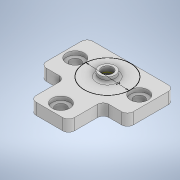
# Autodesk Inventor part: Pulley support
Saved by Autodesk Inventor 2022 (Build 260153000, 153)
## iProperties
Created: 2022-03-05
Part Number: Pulley support
Material: Genérico
Document SubType Name: Modeling
Designer: JK
Density: 1 g/cm^3
Appearance: Valor por defecto
Author: JK
Autodesk Inventor part; units mm, degrees
ref_plane "YZ Plane" through (0, 0, 0) normal (1, 0, 0) x (0, 1, 0)
ref_plane "XZ Plane" through (0, 0, 0) normal (0, 1, 0) x (-1, 0, 0)
ref_plane "XY Plane" through (0, 0, 0) normal (0, 0, 1) x (1, 0, 0)
sketch "Boceto1" plane through (0, 0, 0) normal (0, 1, 0) x (-1, 0, 0)
  circle A0 centre (0, 0) radius 12.15
  dimension "d0" = 24.3
  constraints: 1 centre point, 1 coincident
  measures "d0" diameter of A0
extrude "Extrusión1" add sketch "Boceto1" along normal blind 4
sketch "Boceto2" plane through (0, 0, 0) normal (0, -1, 0) x (1, 0, 0)
  line L0 (4.6765, 0) -> (2.3383, -4.05)
  line L1 (2.3383, -4.05) -> (-2.3383, -4.05)
  line L2 (-2.3383, -4.05) -> (-4.6765, 0)
  line L3 (-4.6765, 0) -> (-2.3383, 4.05)
  line L4 (-2.3383, 4.05) -> (2.3383, 4.05)
  line L5 (2.3383, 4.05) -> (4.6765, 0)
  circle A0 centre (0, 0) radius 4.05
  dimension "d3" = 8.1
  constraints: 12 end point, 2 coincident, 1 centre point, 1 tangent, 13 other
  measures "d3" diameter of A0
extrude "Extrusión2" cut sketch "Boceto2" against normal blind 4
sketch "Boceto3" plane through (0, 4, 0) normal (0, 1, 0) x (1, 0, 0)
  line L0 (2.3383, 4.05) -> (4.6765, 0) projected
  line L1 (4.6765, 0) -> (2.3383, -4.05) projected
  line L2 (2.3383, -4.05) -> (-2.3383, -4.05) projected
  line L3 (-2.3383, -4.05) -> (-4.6765, 0) projected
  line L4 (-4.6765, 0) -> (-2.3383, 4.05) projected
  line L5 (-2.3383, 4.05) -> (2.3383, 4.05) projected
  circle A0 centre (0, 0) radius 12.15 projected
  circle A1 centre (0, 0) radius 2.9
  dimension "d6" = 5.8
  constraints: 1 centre point, 1 coincident
  measures "d6" diameter of A1
extrude "Extrusión3" add sketch "Boceto3" along normal blind 2 contours L0 L1 L2 L3 L4 L5 | A0
sketch "Boceto4" plane through (0, 6, 0) normal (0, 1, 0) x (1, 0, 0)
  circle A0 centre (0, 0) radius 4.2
  circle A1 centre (0, 0) radius 2.9 projected
  dimension "d9" = 8.4
  constraints: 1 centre point, 1 coincident
  measures "d9" diameter of A0
extrude "Extrusión4" add sketch "Boceto4" along normal blind 2.8
fillet "Empalme1" radius 1.3 1 edges at (-4.2, 6, 0)
sketch "Boceto5" plane through (0, 6, 0) normal (0, 1, 0) x (1, 0, 0)
  line L0 (-22.7, -12.15) -> (22.7, -12.15)
  line L1 (22.7, -12.15) -> (22.7, 12.15)
  line L2 (22.7, 12.15) -> (-22.7, 12.15)
  line L3 (-22.7, 12.15) -> (-22.7, -12.15)
  circle A0 centre (0, 0) radius 2.9 projected
  line L4 (-22.7, -12.15) -> (22.7, 12.15) construction
  line L5 (22.7, -12.15) -> (-22.7, 12.15) construction
  circle A1 centre (0, 0) radius 12.15 projected
  point P0 (0, -12.15)
  point P1 (0, 12.15)
  dimension "d13" = 45.4
  constraints: 12 end point, 2 midpoint, 2 parallel, 1 horizontal, 1 perpendicular, 1 tangent
  measures "d13" distance of L1.end L2.end
extrude "Extrusión5" add sketch "Boceto5" against normal up to surface (6 mm away) contours L3 L2 A1 L0 | A1 L2 L1 L0
sketch "Boceto6" plane through (0, 6, 0) normal (0, 1, 0) x (1, 0, 0)
  circle A0 centre (-16.7, 0) radius 2.7
  circle A1 centre (16.7, 0) radius 2.7
  line L0 (-22.7, 12.15) -> (-22.7, -12.15) projected
  line L1 (22.7, -12.15) -> (22.7, 12.15) projected
  point P0 (0, 0)
  dimension "d16" = 5.4
  dimension "d17" = 6
  dimension "d18" = 6
  constraints: 2 centre point, 1 equal radius
  measures "d16" diameter of A0
  measures "d17" distance from line of L0 A0.centre
  measures "d18" distance from line of L1 A1.centre
extrude "Extrusión6" cut sketch "Boceto6" against normal through all
fillet "Empalme2" radius 3 4 edges at (-22.7, 3, 12.15) (22.7, 3, 12.15) (-22.7, 3, -12.15) (22.7, 3, -12.15)
sketch "Boceto7" plane through (0, 6, 0) normal (0, 1, 0) x (1, 0, 0)
  line L0 (-10, 30.2) -> (10, 30.2)
  line L1 (10, 30.2) -> (10, -30.2)
  line L2 (10, -30.2) -> (-10, -30.2)
  line L3 (-10, -30.2) -> (-10, 30.2)
  line L4 (-10, 30.2) -> (10, -30.2) construction
  line L5 (10, 30.2) -> (-10, -30.2) construction
  line L6 (-19.7, -12.15) -> (19.7, -12.15) projected
  circle A0 centre (0, -24.2) radius 2.7
  circle A1 centre (0, 0) radius 21.5
  point P0 (10, -12.15)
  point P1 (-10, -12.15)
  dimension "d22" = 20
  dimension "d24" = 5.4
  dimension "d25" = 6
  dimension "d29" = 43
  constraints: 12 end point, 3 midpoint, 2 centre point, 2 parallel, 1 coincident, 1 horizontal, 1 perpendicular, 1 tangent, 1 vertical alignment
  measures "d22" distance between parallel lines of L3 L1
  measures "d24" diameter of A0
  measures "d25" distance from line of L2 A0.centre
  measures "d29" diameter of A1
extrude "Extrusión7" add sketch "Boceto7" against normal up to surface (6 mm away) contours L6 L1 A1 L3 | A1 L1 L2 L3 picked at (0, -15.2667)
fillet "Empalme3" radius 3 4 edges at (-10, 3, 12.15) (-10, 3, 30.2) (10, 3, 30.2) (10, 3, 12.15)
sketch "Boceto9" plane through (0, 6, 0) normal (0, 1, 0) x (1, 0, 0)
  circle A0 centre (16.7, 0) radius 2.7 projected
  circle A1 centre (16.7, 0) radius 4.65
  circle A2 centre (-16.7, 0) radius 2.7 projected
  circle A3 centre (-16.7, 0) radius 4.65
  circle A4 centre (0, -24.2) radius 2.7 projected
  circle A5 centre (0, -24.2) radius 4.65
  point P0 (0, 0)
  dimension "d30" = 9.3
  constraints: 3 centre point, 3 coincident, 2 equal radius
  measures "d30" diameter of A1
extrude "Extrusión8" cut sketch "Boceto9" against normal blind 2 contours A0 | A1 | A2 | A3 | A4 | A5
sketch "Boceto10" plane through (0, 6, 0) normal (0, 1, 0) x (1, 0, 0)
  circle A0 centre (0, 0) radius 2.9 projected
  circle A1 centre (0, 0) radius 12
  dimension "d33" = 24
  constraints: 1 centre point, 1 coincident
  measures "d33" diameter of A1
